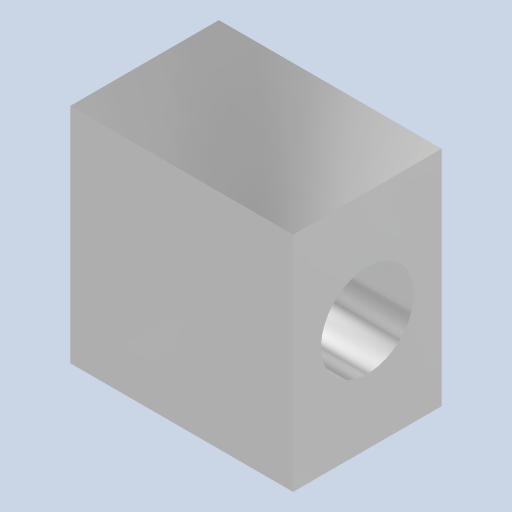
# Autodesk Inventor part: compressionSpacer
Saved by Autodesk Inventor 2023 (Build 270158030, 158C)
## iProperties
Created: 2023-01-21
Part Number: compressionSpacer
Material: Aluminum 6061
Document SubType Name: Modeling
Designer: kumpu
Density: 2.7 g/cm^3
Appearance: Aluminum - Flat
Author: kumpu
Autodesk Inventor part; units mm, degrees
ref_plane "YZ Plane" through (0, 0, 0) normal (1, 0, 0) x (0, 1, 0)
ref_plane "XZ Plane" through (0, 0, 0) normal (0, 1, 0) x (-1, 0, 0)
ref_plane "XY Plane" through (0, 0, 0) normal (0, 0, 1) x (1, 0, 0)
sketch "Sketch1" plane through (0, 0, 0) normal (1, 0, 0) x (0, 1, 0)
  line L0 (9.525, 6.35) -> (-9.525, 6.35)
  line L1 (-9.525, 6.35) -> (-9.525, -6.35)
  line L2 (-9.525, -6.35) -> (9.525, -6.35)
  line L3 (9.525, -6.35) -> (9.525, 6.35)
  line L4 (9.525, 6.35) -> (-9.525, -6.35) construction
  line L5 (-9.525, 6.35) -> (9.525, -6.35) construction
  circle A0 centre (0, 0) radius 3.9688
  dimension "d0" = 7.9375
  dimension "d1" = 19.05
  dimension "d2" = 12.7
  constraints: 12 end point, 2 midpoint, 2 parallel, 1 centre point, 1 coincident, 1 horizontal, 1 perpendicular
  measures "d0" diameter of A0
  measures "d1" distance of L1.end L2.end
  measures "d2" distance of L2.end L0.start
extrude "Extrusion1" add sketch "Sketch1" along normal mid plane 19.05
body "Solid1"
